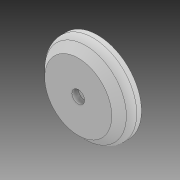
# Autodesk Inventor part: Winder_drivegear
Saved by Autodesk Inventor 2020 (Build 240168000, 168)
## iProperties
Created: 2021-03-13
Part Number: Winder_drivegear
Material: Generic
Document SubType Name: Modeling
Designer: DDeGo
Density: 1 g/cm^3
Appearance: Default
Author: DDeGo
Autodesk Inventor part; units mm, degrees
ref_plane "YZ Plane" through (0, 0, 0) normal (1, 0, 0) x (0, 1, 0)
ref_plane "XZ Plane" through (0, 0, 0) normal (0, 1, 0) x (-1, 0, 0)
ref_plane "XY Plane" through (0, 0, 0) normal (0, 0, 1) x (1, 0, 0)
sketch "Sketch1" plane through (0, 0, 0) normal (1, 0, 0) x (0, 1, 0)
  line L0 (0, 0) -> (0, 7.5)
  line L1 (0, 7.5) -> (2.45, 7.5) construction
  line L2 (2.45, 7.5) -> (2.45, 5)
  line L3 (2.45, 5) -> (4.5, 5)
  line L4 (4.5, 5) -> (4.5, 0)
  line L5 (4.5, 0) -> (0, 0) construction
  line L6 (8.9, 0) -> (8.6, -1.6)
  line L7 (8.6, -1.6) -> (7.4, -1.6)
  line L8 (7.4, -1.6) -> (7.1, 0)
  line L9 (7.1, 0) -> (8.9, 0) construction
  line L10 (17, 0) -> (17, 3.5)
  line L11 (13, 7.5) -> (4.45, 7.5)
  line L12 (4.45, 7.5) -> (2.45, 7.5)
  line L13 (4.5, 0) -> (7.1, 0)
  line L14 (8.9, 0) -> (17, 0)
  line L15 (17, 3.5) -> (13, 7.5)
  point P0 (17, 7.5)
  point P1 (8, 0)
  dimension "d0" = 2.45
  dimension "d3" = 5
  dimension "d4" = 2.5
  dimension "d5" = 4.5
  dimension "d6" = 8
  dimension "d7" = 1.2
  dimension "d8" = 1.8
  dimension "d9" = 1.6
  dimension "d11" = 4
  dimension "d12" = 4
  dimension "d14" = 17
  constraints: 32 end point, 7 perpendicular, 3 point on line, 1 collinear, 1 equal length, 1 horizontal, 1 midpoint, 1 vertical
  measures "d0" distance between parallel lines of L0 L2
  measures "d3" distance between parallel lines of L5 L3
  measures "d4" distance between parallel lines of L3 L11
  measures "d5" distance between parallel lines of L0 L4
  measures "d6" distance from line of L0 point (8, 0)
  measures "d7" distance of L6.end L7.end
  measures "d8" distance of L8.end L6.start
  measures "d9" distance between parallel lines of L9 L7
  measures "d11" distance of L10.end point (17, 7.5)
  measures "d12" distance of L11.start point (17, 7.5)
  measures "d14" distance between parallel lines of L0 L10
revolve "Revolution1" add sketch "Sketch1" angle 360 about axis through (0, 0, 0) along (0, 0, 1)
sketch "Sketch2" plane through (0, 0, 0) normal (0, 0, -1) x (-1, 0, 0)
  circle A0 centre (0, 0) radius 7.1 projected
  line L0 (0, 0) -> (0, 13) construction
  circle A1 centre (0, 13) radius 1.85
  point P0 (0, 0)
  dimension "d15" = 13
  dimension "d16" = 3.7
  constraints: 2 end point, 1 centre point, 1 coincident, 1 vertical
  measures "d15" distance of L0.start L0.end
  measures "d16" diameter of A1
extrude "Extrusion1" add sketch "Sketch2" along normal blind 1.4 contours A1
chamfer "Chamfer1" distance 0.5 angle 45 1 edges at (1.85, 13, -1.4)
fillet "Fillet1" radius 1 1 edges at (1.85, 13, -0.9)
pattern_circular "Circular Pattern1" count 12 over 360 about axis through (0, 0, 2.5) along (0, 0, -1) of "Extrusion1", "Chamfer1", "Fillet1"
fillet "Fillet2" radius 0.5 2 edges at (0, -8.6, -1.6) (0, -7.4, -1.6)
fillet "Fillet2" radius 4 1 edges at (0, -17, 3.5)
equation "\"d12\" = d11"
body "Solid1"
